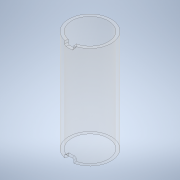
# Autodesk Inventor part: HSI
Saved by Autodesk Inventor 2022 (Build 260153000, 153)
## iProperties
Created: 2022-03-30
Part Number: HSI
Material: Polycarbonate, Clear
Document SubType Name: Modeling
Designer: RNG3nius
Density: 1.2 g/cm^3
Appearance: Polycarbonate - Clear
Mass: 74.1116 g
Surface Area: 571.047 cm^2
Volume: 61.7597 cm^3
Author: RNG3nius
Autodesk Inventor part; units mm, degrees
ref_plane "YZ Plane" through (0, 0, 0) normal (1, 0, 0) x (0, 1, 0)
ref_plane "XZ Plane" through (0, 0, 0) normal (0, 1, 0) x (-1, 0, 0)
ref_plane "XY Plane" through (0, 0, 0) normal (0, 0, 1) x (1, 0, 0)
sketch "Sketch5" plane through (0, 0, 0) normal (0, 1, 0) x (-1, 0, 0)
  circle A0 centre (0, 0) radius 28.8
  circle A1 centre (0, 0) radius 24.8
  dimension "d26" = 57.6
  dimension "d27" = 49.6
  constraints: 2 centre point, 2 coincident
  measures "d26" diameter of A0
  measures "d27" diameter of A1
extrude "Extrusion3" add sketch "Sketch5" along normal blind 138.4
sketch "Sketch6" plane through (0, 0, 0) normal (1, 0, 0) x (0, 1, 0)
  line L0 (138.4, 24.8) -> (0, 24.8) projected
  line L1 (0, 28.8) -> (138.4, 28.8) projected
  line L2 (0, -28.8) -> (0, 28.8) projected
  line L3 (0, 28.8) -> (5.6, 28.8)
  line L4 (5.6, 28.8) -> (5.6, 24.8)
  line L5 (5.6, 24.8) -> (0, 24.8)
  line L6 (0, 24.8) -> (0, 28.8)
  line L7 (138.4, -28.8) -> (138.4, 28.8) projected
  line L8 (138.4, 28.8) -> (132.8, 28.8)
  line L9 (132.8, 28.8) -> (132.8, 24.8)
  line L10 (132.8, 24.8) -> (138.4, 24.8)
  line L11 (138.4, 24.8) -> (138.4, 28.8)
  line L12 (-27.68, 0) -> (166.08, 0) projected
  point P0 (0, 0)
  dimension "d31" = 5.6
  dimension "d32" = 4
  dimension "d33" = 5.6
  dimension "d34" = 4
  constraints: 16 end point, 4 parallel, 2 horizontal, 2 perpendicular
  measures "d31" distance of L4.end L5.end
  measures "d32" distance of L3.end L4.end
  measures "d33" distance of L10.end L9.end
  measures "d34" distance of L9.end L8.end
revolve "Revolution2" cut sketch "Sketch6" angle 12.51 about axis through (0, -10, 0) along (0, 1, 0) and the other way 12.51 contours L0 L9 L1 L7 | L0 L2 L1 L4
fillet "Fillet3" radius 2 4 edges at (-5.8051, 5.6, 26.1637) (5.8051, 5.6, 26.1637) (-5.8051, 132.8, 26.1637) (5.8051, 132.8, 26.1637)
body "Solid2"
